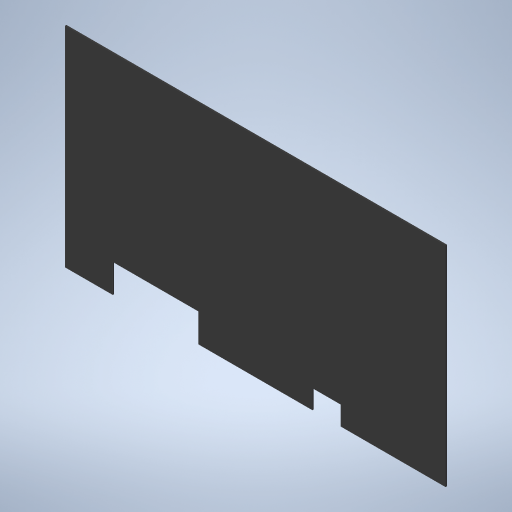
# Autodesk Inventor part: Top Intake Poly (Sponsor Panel)
Saved by Autodesk Inventor 2023 (Build 270158000, 158)
## iProperties
Created: 2024-02-16
Part Number: Top Intake Poly (Sponsor Panel)
Material: Generic
Document SubType Name: Modeling
Designer: Robodox
Density: 1 g/cm^3
Appearance: Default
Author: Robodox
Autodesk Inventor part; units mm, degrees
ref_plane "YZ Plane" through (0, 0, 0) normal (1, 0, 0) x (0, 1, 0)
ref_plane "XZ Plane" through (0, 0, 0) normal (0, 1, 0) x (-1, 0, 0)
ref_plane "XY Plane" through (0, 0, 0) normal (0, 0, 1) x (1, 0, 0)
sketch "Sketch1" plane through (0, 0, 0) normal (0, 0, 1) x (1, 0, 0)
  line L0 (-125.8778, 76.6863) -> (128.1222, 76.6863)
  line L1 (128.1222, 76.6863) -> (128.1222, -63.0137)
  line L2 (128.1222, -63.0137) -> (-125.8778, -63.0137)
  line L3 (-125.8778, -63.0137) -> (-125.8778, 76.6863)
  line L4 (-125.8778, -63.0137) -> (-94.1278, -63.0137)
  line L5 (-94.1278, -63.0137) -> (-94.1278, -43.9637)
  line L6 (-94.1278, -43.9637) -> (-36.9778, -43.9637)
  line L7 (-36.9778, -43.9637) -> (-36.9778, -63.0137)
  line L8 (128.1222, -63.0137) -> (58.2722, -63.0137)
  line L9 (58.2722, -63.0137) -> (58.2722, -50.3137)
  line L10 (58.2722, -50.3137) -> (39.2222, -50.3137)
  line L11 (39.2222, -50.3137) -> (39.2222, -63.0137)
  point P0 (0, 0)
  dimension "d0" = 254
  dimension "d1" = 139.7
  dimension "d6" = 31.75
  dimension "d7" = 19.05
  dimension "d8" = 57.15
  dimension "d9" = 69.85
  dimension "d10" = 12.7
  dimension "d11" = 19.05
  constraints: 24 end point, 7 perpendicular, 4 point on line, 2 parallel, 1 horizontal
  measures "d0" distance of L0.start L0.end
  measures "d1" distance of L0.end L1.end
  measures "d6" distance of L2.end L4.end
  measures "d7" distance of L4.end L5.end
  measures "d8" distance of L5.end L6.end
  measures "d9" distance of L1.end L8.end
  measures "d10" distance of L8.end L9.end
  measures "d11" distance of L9.end L10.end
extrude "Extrusion3" add sketch "Sketch1" along normal blind 0.7937 contours L0 L1 L2 L9 L10 L11 L7 L6 L5 L3
body "Solid3"
